joint (Autodesk Fusion 360 design; units mm, degrees)
Autodesk Fusion 360 part; units mm, degrees
sketch "Sketch1" plane through (0, 0, 0) normal (0, 0, 1) x (1, 0, 0)
  circle A0 centre (0, 0) radius 18.925
  circle A1 centre (0, 0) radius 7.5
  dimension "d1" = 37.85
  dimension "d2" = 15
  constraint coincident A0.centre A1.centre
  measures "d1" diameter of A0
  measures "d2" diameter of A1
extrude "Extrude1" add sketch "Sketch1" along normal blind 40 contours A0 | A1
extrude "Extrude2" add sketch "Sketch1" against normal blind 16.846 contours A1
extrude "Extrude3" add sketch "Sketch1" along normal blind 16.846 from surface at 40 contours A1
delete_face "DeleteFace1" 1 faces at (7.4907, -0.3738, -11.2307)
ref_plane "WorkPlane1" through (0, 0, 20) normal (0, 0, 1) x (1, 0, 0)
sketch "Sketch2" plane through (0, 0, 56.846) normal (0, 0, 1) x (-1, 0, 0)
  circle A0 centre (0, 0) radius 7.5
  line L0 (0.75, 2) -> (-0.75, 2)
  line L1 (-0.75, 2) -> (-0.75, -2)
  line L2 (-0.75, -2) -> (0.75, -2)
  line L3 (0.75, -2) -> (0.75, 2)
  line L4 (0.75, 2) -> (-0.75, -2) construction
  line L5 (-0.75, 2) -> (0.75, -2) construction
  dimension "d10" = 1.5
  dimension "d11" = 4
  constraint horizontal L0
  constraint perpendicular L0 L1
  constraint parallel L0 L2
  constraint parallel L1 L3
  constraint coincident L4 A0.centre
  constraint coincident L5 A0.centre
  constraint coincident A0.centre origin
  measures "d10" distance of L1.end L2.end
  measures "d11" distance of L0.end L1.end
extrude "Extrude4" cut sketch "Sketch2" against normal blind 4 contours L0 L1 L2 L3
chamfer "Chamfer1" distance 1 angle 45 2 edges at (0, 2, 56.846) (0, -2, 56.846)
chamfer "Chamfer2" distance 0.2 angle 45 1 edges at (-6.9925, -2.7121, 56.846)
mirror "Mirror1" about plane through (0, 0, 20) normal (0, 0, 1) of 10 faces at (2.9333, 0, 56.846) (-0.25, -2.6667, 56.5127) (6.985, 2.5423, 56.7127) (-0.75, 0.6667, 54.846) (-0.25, -2, 54.846) (0.75, -0.6667, 54.846) (0.25, -0.6667, 52.846) (0.25, 2.6667, 56.5127) (0.25, 2, 54.846) (7.4907, -0.3738, 51.0973)
equation "d1 = 18.925 * 2 mm"
equation "d2 = 7.50 * 2 mm"
